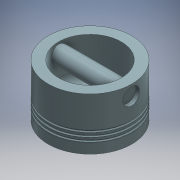
# Autodesk Inventor part: Piston
Saved by Autodesk Inventor 2016 (Build 200138000, 138)
## iProperties
Created: 2017-07-15
Part Number: Piston
Material: Steel, Carbon
Document SubType Name: Modeling
Designer: bobbyl
Density: 7.85 g/cm^3
Appearance: Lead
Mass: 146.659 g
Surface Area: 87.7069 cm^2
Volume: 18.6827 cm^3
Author: bobbyl
Autodesk Inventor part; units mm, degrees
ref_plane "XZ Plane" through (0, 0, 0) normal (0, 1, 0) x (-1, 0, 0)
sketch "Sketch1" plane through (0, 0, 0) normal (0, 0, 1) x (1, 0, 0)
  circle A0 centre (0, 0) radius 20
  dimension "d0" = 40
  constraints: 1 centre point, 1 coincident
  measures "d0" diameter of A0
extrude "Extrusion1" add sketch "Sketch1" along normal blind 25
shell "Shell1" thickness 5 removed faces 1 at (-2.364, 6.2334, 25)
fillet "Fillet1" radius 5 1 edges at (-15, 0, 5)
sketch "Sketch2" plane through (0, 0, 0) normal (1, 0, 0) x (0, 1, 0)
  line L0 (-28, 0) -> (28, 0) projected
  line L1 (0, -5) -> (0, 30) projected
  circle A0 centre (0, 20) radius 4
  line L2 (20, 25) -> (-20, 25) projected
  point P0 (0, 0)
  dimension "d5" = 8
  dimension "d6" = 5
  constraints: 1 centre point, 1 point on line
  measures "d5" diameter of A0
  measures "d6" distance from line of L2 A0.centre
extrude "Extrusion2" add sketch "Sketch2" along normal through all both and the other way through all
ref_plane "Work Plane1" through (18, 0, 0) normal (1, 0, 0) x (0, 1, 0)
sketch "Sketch3" plane through (18, 0, 0) normal (1, 0, 0) x (0, 1, 0)
  spline S0 degree 5 poles (4, 20) (4, 20.475) (3.9296, 20.9492) (3.7887, 21.4163) (3.5746, 21.8668) (3.0962, 22.5531) (2.8791, 22.8072) (2.6286, 23.0458) (2.3433, 23.263) (1.6847, 23.649) (1.3023, 23.8174) (0.8849, 23.938) (0.4453, 24) (-0.4453, 24) (-0.8849, 23.938) (-1.3023, 23.8174) (-1.6847, 23.649) (-2.3433, 23.263) (-2.6286, 23.0458) (-2.8791, 22.8072) (-3.0962, 22.5531) (-3.5746, 21.8668) (-3.7887, 21.4163) (-3.9296, 20.9492) (-4, 20.475) (-4, 19.6437) (-3.9603, 19.2875) (-3.881, 18.9346) (-3.7611, 18.5887) (-3.4806, 18.0102) (-3.3396, 17.7723) (-3.1752, 17.5422) (-2.9865, 17.3225) (-2.4836, 16.839) (-2.1457, 16.5837) (-1.7587, 16.3645) (-1.3265, 16.1959) (-0.4314, 15.9995) (0.0204, 15.9613) (0.4754, 15.9901) (0.9122, 16.0827) (1.662, 16.3427) (1.9854, 16.5006) (2.2787, 16.6866) (2.5408, 16.8939) (3.2793, 17.604) (3.6446, 18.1696) (3.8809, 18.7676) (4, 19.3828) (4, 20) knots 0 0 0 0 0 0 0.108769 0.108769 0.108769 0.108769 0.177598 0.177598 0.177598 0.177598 0.250135 0.250135 0.250135 0.250135 0.322672 0.322672 0.322672 0.322672 0.3915 0.3915 0.3915 0.3915 0.50027 0.50027 0.50027 0.50027 0.581861 0.581861 0.581861 0.581861 0.641459 0.641459 0.641459 0.641459 0.721814 0.721814 0.721814 0.721814 0.794745 0.794745 0.794745 0.794745 0.859101 0.859101 0.859101 0.859101 1 1 1 1 1 1 projected
  point P0 (0, 0)
  dimension "d10" = 0
  constraints: 3 other
extrude "Extrusion3" cut sketch "Sketch3" along normal through all
mirror "Mirror1" about plane through (0, 0, 0) normal (1, 0, 0) of "Extrusion3"
ref_plane "Work Plane2" through (0, 0, 5) normal (0, 0, 1) x (1, 0, 0)
sketch "Sketch4" plane through (0, 0, 5) normal (0, 0, 1) x (1, 0, 0)
  circle A0 centre (0, 0) radius 15 projected
  circle A1 centre (0, 0) radius 20 projected
  circle A2 centre (0, 0) radius 19
  dimension "d14" = 1
  constraints: 1 centre point
  measures "d14" radial gap between concentric circles of A1 A2
extrude "Extrusion4" cut sketch "Sketch4" along normal blind 1 contours A1
pattern_linear "Rectangular Pattern1" count 3 spacing 2 along (0, 0, 1) of "Extrusion4"
body "Solid1"
